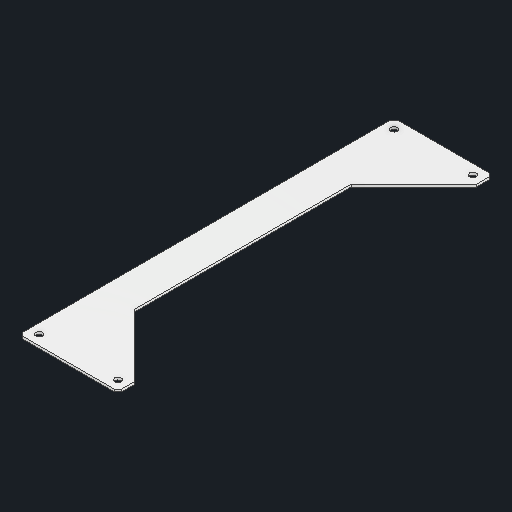
# Autodesk Inventor part: Ramp
Saved by Autodesk Inventor 2025 (Build 290162000, 162)
## iProperties
Created: 2024-12-22
Part Number: Ramp
Material: Acetal Resin, White
Document SubType Name: Modeling
Designer: Averey Ku
Density: 1.425 g/cm^3
Appearance: Smooth - White
Author: Averey Ku
Autodesk Inventor part; units mm, degrees
ref_plane "YZ Plane" through (0, 0, 0) normal (1, 0, 0) x (0, 1, 0)
ref_plane "XZ Plane" through (0, 0, 0) normal (0, 1, 0) x (-1, 0, 0)
ref_plane "XY Plane" through (0, 0, 0) normal (0, 0, 1) x (1, 0, 0)
sketch "Sketch1" plane through (0, 0, 0) normal (0, 1, 0) x (-1, 0, 0)
  circle A0 centre (-26.7822, 116.9636) radius 2.1844
  circle A1 centre (24.0178, 116.9636) radius 2.1844
  circle A2 centre (24.0178, -111.6364) radius 2.1844
  circle A3 centre (-26.7822, -111.6364) radius 2.1844
  line L0 (-33.1322, -107.5724) -> (-33.1322, -115.7004)
  line L1 (-33.1322, -115.7004) -> (-30.8462, -117.9864)
  line L2 (-30.8462, -117.9864) -> (-22.7182, -117.9864)
  line L3 (19.9538, -117.9864) -> (28.0818, -117.9864)
  line L4 (28.0818, -117.9864) -> (30.3678, -115.7004)
  line L5 (30.3678, -115.7004) -> (30.3678, 112.8996)
  line L6 (30.3678, 112.8996) -> (30.3678, 121.0276)
  line L7 (30.3678, 121.0276) -> (28.0818, 123.3136)
  line L8 (28.0818, 123.3136) -> (19.9538, 123.3136)
  line L9 (-22.7182, 123.3136) -> (-30.8462, 123.3136)
  line L10 (-30.8462, 123.3136) -> (-33.1322, 121.0276)
  line L11 (-33.1322, 121.0276) -> (-33.1322, 112.8996)
  line L12 (-33.1322, 112.8996) -> (-26.8076, 106.575)
  line L13 (0.9292, 78.8382) -> (7.2538, 72.5136)
  line L14 (-30.8462, 123.3136) -> (28.0818, 123.3136)
  line L15 (0.9292, 78.8382) -> (-26.8076, 106.575)
  line L16 (7.2538, 72.5136) -> (7.2538, -67.1864)
  line L17 (7.2538, -67.1864) -> (-33.1322, -107.5724)
  line L18 (19.9538, -117.9864) -> (-22.7182, -117.9864)
  point P0 (0, 0)
  constraints: 38 end point, 4 centre point, 2 vertical, 1 collinear, 1 horizontal, 1 perpendicular
extrude "Extrusion1" add sketch "Sketch1" along normal blind 1.5875
body "Solid1"
